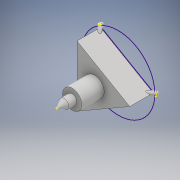
# Autodesk Inventor part: 噴頭
Saved by Autodesk Inventor 2017 (Build 210142000, 142)
## iProperties
Part Number: 噴頭
Material: 一般
Document SubType Name: Modeling
Designer: Brian
Density: 1 g/cm^3
Appearance: 預設
Author: Brian
Autodesk Inventor part; units mm, degrees
ref_plane "YZ Plane" through (0, 0, 0) normal (1, 0, 0) x (0, 1, 0)
ref_plane "XZ Plane" through (0, 0, 0) normal (0, 1, 0) x (-1, 0, 0)
sketch "草圖1" plane through (0, 0, 0) normal (0, 0, 1) x (1, 0, 0)
  line L0 (0, 0) -> (2, 3.25)
  line L1 (2, 3.25) -> (2, 6.6667)
  line L2 (2, 6.6667) -> (4.1026, 6.6667)
  line L3 (4.1026, 6.6667) -> (4.1026, 16.25)
  line L4 (4.1026, 16.25) -> (0, 16.25)
  line L5 (0, 16.25) -> (0, 0)
  dimension "d0" = 2
  constraints: 12 end point, 4 perpendicular, 1 point on line, 1 vertical
  measures "d0" distance between parallel lines of L5 L1
revolve "迴轉1" add sketch "草圖1" angle 360 about axis through (0, 16.25, 0) along (0, -1, 0)
sketch "草圖2" plane through (0, 16.25, 0) normal (0, 1, 0) x (1, 0, 0)
  line L0 (15, 0) -> (-7.5, -12.9904)
  line L1 (-7.5, -12.9904) -> (-7.5, 12.9904)
  line L2 (-7.5, 12.9904) -> (15, 0)
  circle A0 centre (0, 0) radius 2 projected
  dimension "d32" = 15
  constraints: 6 end point, 1 coincident, 7 other
  measures "d32" distance of A0.centre L0.start
extrude "擠出1" add sketch "草圖2" along normal blind 10 contours L0 L1 L2 | A0
scale "比例1" factors (3, 3, 3) then translate (-7.5, -52.5, -12.9904) bodies 1
ref_plane "工作平面3" through (37.5, -3.75, -12.9904) normal (0, 0, 1) x (0, 1, 0)
sketch "草圖5" plane through (37.5, -3.75, -12.9904) normal (0, 0, 1) x (0, 1, 0)
  line L0 (33.7678, -3.7678) -> (21.5899, 8.4101)
  line L1 (21.5899, 8.4101) -> (23.3577, 10.1778)
  line L2 (23.3577, 10.1778) -> (35.5355, -2)
  line L3 (35.5355, -2) -> (33.7678, -3.7678)
  line L4 (0, 0) -> (30, 0) projected
  point P0 (3.75, 37.5)
  point P1 (32, -2)
  dimension "d22" = 2.5
  dimension "d28" = 2.5
  dimension "d29" = 2
  dimension "d31" = 135
  constraints: 8 end point, 2 parallel, 2 point on line, 1 perpendicular
  measures "d22" distance of L0.end L1.end
  measures "d28" distance of L0.start point (32, -2)
  measures "d29" distance from line of L4 point (32, -2)
  measures "d31" angle of L4 L0
revolve "迴轉2" add sketch "草圖5" angle 360 about axis through (41.2678, 30.0178, -12.9904) along (-0.7071068, -0.7071068, 0)
fillet "圓角2" radius 2.5 1 edges at (43.0355, 28.25, -12.9904)
pattern_circular "環形陣列2" count 3 over 360 about axis through (-7.5, -18.125, -12.9904) along (0, -1, 0) of "迴轉2", "圓角2"
sketch "草圖6" plane through (-30, 26.25, 22.8185) normal (0, 1, 0) x (1, 0, 0)
  arc A0 (-3.1651, -3.6443) -> (1.1651, -6.1443) centre (-1, -4.8943) ccw projected
  arc A1 (1.1651, 77.7621) -> (-3.1651, 75.2621) centre (-1, 76.5121) ccw projected
  arc A2 (69.5, 33.3089) -> (69.5, 38.3089) centre (69.5, 35.8089) ccw projected
  line L0 (-1, -4.8943) -> (-1, 76.5121)
  line L1 (-1, 76.5121) -> (69.5, 35.8089)
  line L2 (0, 74.78) -> (4.3301, 72.28) projected
  ellipse E0 centre (-1, -4.8943) end of major axis (-3.1651, -3.6443) minor radius 1.7678 projected
  line L3 (69.5, 35.8089) -> (-1, -4.8943)
  circle A3 centre (22.5, 35.8089) radius 6 projected
  circle A4 centre (22.5, 35.8089) radius 47
  point P0 (30, 22.8185)
  point P1 (2.7386, 73.1989)
  constraints: 6 end point, 1 coincident, 1 parallel, 1 vertical, 4 other
